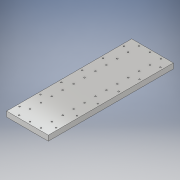
# Autodesk Inventor part: AlTop
Saved by Autodesk Inventor 2019.4 (Build 234330000, 330)
## iProperties
Created: 2020-04-27
Part Number: AlTop
Material: Generic
Document SubType Name: Modeling
Designer: Ed
Density: 1 g/cm^3
Appearance: Default
Author: Ed
Autodesk Inventor part; units mm, degrees
ref_plane "YZ Plane" through (0, 0, 0) normal (1, 0, 0) x (0, 1, 0)
ref_plane "XZ Plane" through (0, 0, 0) normal (0, 1, 0) x (-1, 0, 0)
ref_plane "XY Plane" through (0, 0, 0) normal (0, 0, 1) x (1, 0, 0)
sketch "Sketch1" plane through (0, 0, 0) normal (0, 1, 0) x (-1, 0, 0)
  arc A0 (49.1631, 298.6655) -> (49.149, 298.45) centre (50.8, 298.45) ccw
  arc A1 (49.149, 298.45) -> (52.3947, 298.0227) centre (50.8, 298.45) ccw
  arc A2 (52.3947, 298.0227) -> (52.451, 298.45) centre (50.8, 298.45) ccw
  arc A3 (52.451, 298.45) -> (49.2053, 298.8773) centre (50.8, 298.45) ccw
  arc A4 (49.2053, 298.8773) -> (49.1631, 298.6655) centre (50.8, 298.45) ccw
  arc A5 (22.7572, 297.5315) -> (22.9626, 297.2813) centre (24.13, 298.4487) ccw
  arc A6 (22.9626, 297.2813) -> (25.781, 298.4487) centre (24.13, 298.4487) ccw
  arc A7 (25.781, 298.4487) -> (22.5353, 298.876) centre (24.13, 298.4487) ccw
  arc A8 (22.5353, 298.876) -> (22.479, 298.4487) centre (24.13, 298.4487) ccw
  arc A9 (22.479, 298.4487) -> (22.7572, 297.5315) centre (24.13, 298.4487) ccw
  arc A10 (7.7798, 278.5745) -> (8.001, 279.4) centre (6.35, 279.4) ccw
  arc A11 (8.001, 279.4) -> (7.5174, 280.5674) centre (6.35, 279.4) ccw
  arc A12 (7.5174, 280.5674) -> (6.35, 281.051) centre (6.35, 279.4) ccw
  arc A13 (6.35, 281.051) -> (5.1826, 280.5674) centre (6.35, 279.4) ccw
  arc A14 (5.1826, 280.5674) -> (4.699, 279.4) centre (6.35, 279.4) ccw
  arc A15 (4.699, 279.4) -> (7.7798, 278.5745) centre (6.35, 279.4) ccw
  arc A16 (23.8079, 270.275) -> (24.13, 270.2433) centre (24.13, 271.8943) ccw
  arc A17 (24.13, 270.2433) -> (25.781, 271.8943) centre (24.13, 271.8943) ccw
  arc A18 (25.781, 271.8943) -> (23.3045, 273.3241) centre (24.13, 271.8943) ccw
  arc A19 (23.3045, 273.3241) -> (22.7002, 272.7198) centre (24.13, 271.8943) ccw
  arc A20 (22.7002, 272.7198) -> (22.479, 271.8943) centre (24.13, 271.8943) ccw
  arc A21 (22.479, 271.8943) -> (23.8079, 270.275) centre (24.13, 271.8943) ccw
  arc A22 (22.7002, 244.5144) -> (25.781, 245.3399) centre (24.13, 245.3399) ccw
  arc A23 (25.781, 245.3399) -> (24.4521, 246.9591) centre (24.13, 245.3399) ccw
  arc A24 (24.4521, 246.9591) -> (23.7027, 246.9346) centre (24.13, 245.3399) ccw
  arc A25 (23.7027, 246.9346) -> (22.479, 245.3399) centre (24.13, 245.3399) ccw
  arc A26 (22.479, 245.3399) -> (22.7002, 244.5144) centre (24.13, 245.3399) ccw
  arc A27 (7.7798, 227.7745) -> (8.001, 228.6) centre (6.35, 228.6) ccw
  arc A28 (8.001, 228.6) -> (7.5174, 229.7674) centre (6.35, 228.6) ccw
  arc A29 (7.5174, 229.7674) -> (6.35, 230.251) centre (6.35, 228.6) ccw
  arc A30 (6.35, 230.251) -> (4.699, 228.6) centre (6.35, 228.6) ccw
  arc A31 (4.699, 228.6) -> (7.7798, 227.7745) centre (6.35, 228.6) ccw
  arc A32 (23.7027, 217.1907) -> (25.781, 218.7854) centre (24.13, 218.7854) ccw
  arc A33 (25.781, 218.7854) -> (23.7027, 220.3802) centre (24.13, 218.7854) ccw
  arc A34 (23.7027, 220.3802) -> (22.8202, 219.7905) centre (24.13, 218.7854) ccw
  arc A35 (22.8202, 219.7905) -> (22.479, 218.7854) centre (24.13, 218.7854) ccw
  arc A36 (22.479, 218.7854) -> (23.7027, 217.1907) centre (24.13, 218.7854) ccw
  arc A37 (22.7002, 191.4055) -> (25.781, 192.231) centre (24.13, 192.231) ccw
  arc A38 (25.781, 192.231) -> (24.4521, 193.8503) centre (24.13, 192.231) ccw
  arc A39 (24.4521, 193.8503) -> (23.7027, 193.8258) centre (24.13, 192.231) ccw
  arc A40 (23.7027, 193.8258) -> (22.479, 192.231) centre (24.13, 192.231) ccw
  arc A41 (22.479, 192.231) -> (22.7002, 191.4055) centre (24.13, 192.231) ccw
  arc A42 (7.5174, 176.6326) -> (8.001, 177.8) centre (6.35, 177.8) ccw
  arc A43 (8.001, 177.8) -> (7.7228, 178.7172) centre (6.35, 177.8) ccw
  arc A44 (7.7228, 178.7172) -> (6.35, 179.451) centre (6.35, 177.8) ccw
  arc A45 (6.35, 179.451) -> (4.699, 177.8) centre (6.35, 177.8) ccw
  arc A46 (4.699, 177.8) -> (7.5174, 176.6326) centre (6.35, 177.8) ccw
  arc A47 (23.7027, 164.0818) -> (25.781, 165.6766) centre (24.13, 165.6766) ccw
  arc A48 (25.781, 165.6766) -> (24.13, 167.3276) centre (24.13, 165.6766) ccw
  arc A49 (24.13, 167.3276) -> (22.9626, 166.844) centre (24.13, 165.6766) ccw
  arc A50 (22.9626, 166.844) -> (22.479, 165.6766) centre (24.13, 165.6766) ccw
  arc A51 (22.479, 165.6766) -> (23.7027, 164.0818) centre (24.13, 165.6766) ccw
  arc A52 (22.7002, 138.2966) -> (25.781, 139.1221) centre (24.13, 139.1221) ccw
  arc A53 (25.781, 139.1221) -> (24.4521, 140.7414) centre (24.13, 139.1221) ccw
  arc A54 (24.4521, 140.7414) -> (24.3723, 140.7553) centre (24.13, 139.1221) ccw
  arc A55 (24.3723, 140.7553) -> (24.13, 140.7731) centre (24.13, 139.1221) ccw
  arc A56 (24.13, 140.7731) -> (22.479, 139.1221) centre (24.13, 139.1221) ccw
  arc A57 (22.479, 139.1221) -> (22.7002, 138.2966) centre (24.13, 139.1221) ccw
  arc A58 (7.5174, 125.8326) -> (8.001, 127) centre (6.35, 127) ccw
  arc A59 (8.001, 127) -> (7.7228, 127.9172) centre (6.35, 127) ccw
  arc A60 (7.7228, 127.9172) -> (6.35, 128.651) centre (6.35, 127) ccw
  arc A61 (6.35, 128.651) -> (4.699, 127) centre (6.35, 127) ccw
  arc A62 (4.699, 127) -> (7.5174, 125.8326) centre (6.35, 127) ccw
  arc A63 (23.7027, 110.973) -> (25.781, 112.5677) centre (24.13, 112.5677) ccw
  arc A64 (25.781, 112.5677) -> (24.13, 114.2187) centre (24.13, 112.5677) ccw
  arc A65 (24.13, 114.2187) -> (22.9626, 113.7352) centre (24.13, 112.5677) ccw
  arc A66 (22.9626, 113.7352) -> (22.479, 112.5677) centre (24.13, 112.5677) ccw
  arc A67 (22.479, 112.5677) -> (23.7027, 110.973) centre (24.13, 112.5677) ccw
  arc A68 (22.5353, 85.586) -> (25.781, 86.0133) centre (24.13, 86.0133) ccw
  arc A69 (25.781, 86.0133) -> (24.4521, 87.6326) centre (24.13, 86.0133) ccw
  arc A70 (24.4521, 87.6326) -> (24.3723, 87.6464) centre (24.13, 86.0133) ccw
  arc A71 (24.3723, 87.6464) -> (24.13, 87.6643) centre (24.13, 86.0133) ccw
  arc A72 (24.13, 87.6643) -> (22.479, 86.0133) centre (24.13, 86.0133) ccw
  arc A73 (22.479, 86.0133) -> (22.5353, 85.586) centre (24.13, 86.0133) ccw
  arc A74 (7.5174, 75.0326) -> (8.001, 76.2) centre (6.35, 76.2) ccw
  arc A75 (8.001, 76.2) -> (7.8753, 76.8318) centre (6.35, 76.2) ccw
  arc A76 (7.8753, 76.8318) -> (6.35, 77.851) centre (6.35, 76.2) ccw
  arc A77 (6.35, 77.851) -> (4.699, 76.2) centre (6.35, 76.2) ccw
  arc A78 (4.699, 76.2) -> (7.5174, 75.0326) centre (6.35, 76.2) ccw
  arc A79 (23.7027, 57.8641) -> (25.781, 59.4589) centre (24.13, 59.4589) ccw
  arc A80 (25.781, 59.4589) -> (24.13, 61.1099) centre (24.13, 59.4589) ccw
  arc A81 (24.13, 61.1099) -> (23.2128, 60.8316) centre (24.13, 59.4589) ccw
  arc A82 (23.2128, 60.8316) -> (22.479, 59.4589) centre (24.13, 59.4589) ccw
  arc A83 (22.479, 59.4589) -> (23.7027, 57.8641) centre (24.13, 59.4589) ccw
  arc A84 (22.5353, 32.4771) -> (25.781, 32.9044) centre (24.13, 32.9044) ccw
  arc A85 (25.781, 32.9044) -> (24.4521, 34.5237) centre (24.13, 32.9044) ccw
  arc A86 (24.4521, 34.5237) -> (24.3723, 34.5376) centre (24.13, 32.9044) ccw
  arc A87 (24.3723, 34.5376) -> (24.13, 34.5554) centre (24.13, 32.9044) ccw
  arc A88 (24.13, 34.5554) -> (22.479, 32.9044) centre (24.13, 32.9044) ccw
  arc A89 (22.479, 32.9044) -> (22.5353, 32.4771) centre (24.13, 32.9044) ccw
  arc A90 (7.1755, 23.9702) -> (8.001, 25.4) centre (6.35, 25.4) ccw
  arc A91 (8.001, 25.4) -> (7.9299, 25.8793) centre (6.35, 25.4) ccw
  arc A92 (7.9299, 25.8793) -> (7.8753, 26.0318) centre (6.35, 25.4) ccw
  arc A93 (7.8753, 26.0318) -> (6.35, 27.051) centre (6.35, 25.4) ccw
  arc A94 (6.35, 27.051) -> (4.699, 25.4) centre (6.35, 25.4) ccw
  arc A95 (4.699, 25.4) -> (7.1755, 23.9702) centre (6.35, 25.4) ccw
  arc A96 (25.7247, 5.9227) -> (25.781, 6.35) centre (24.13, 6.35) ccw
  arc A97 (25.781, 6.35) -> (24.13, 8.001) centre (24.13, 6.35) ccw
  arc A98 (24.13, 8.001) -> (23.2128, 7.7228) centre (24.13, 6.35) ccw
  arc A99 (23.2128, 7.7228) -> (22.479, 6.35) centre (24.13, 6.35) ccw
  arc A100 (22.479, 6.35) -> (25.7247, 5.9227) centre (24.13, 6.35) ccw
  arc A101 (52.4369, 6.1345) -> (52.451, 6.35) centre (50.8, 6.35) ccw
  arc A102 (52.451, 6.35) -> (50.3727, 7.9447) centre (50.8, 6.35) ccw
  arc A103 (50.3727, 7.9447) -> (49.149, 6.35) centre (50.8, 6.35) ccw
  arc A104 (49.149, 6.35) -> (52.3947, 5.9227) centre (50.8, 6.35) ccw
  arc A105 (52.3947, 5.9227) -> (52.4369, 6.1345) centre (50.8, 6.35) ccw
  arc A106 (78.7462, 7.3974) -> (77.0427, 7.9447) centre (77.47, 6.35) ccw
  arc A107 (77.0427, 7.9447) -> (75.819, 6.35) centre (77.47, 6.35) ccw
  arc A108 (75.819, 6.35) -> (79.121, 6.35) centre (77.47, 6.35) ccw
  arc A109 (79.121, 6.35) -> (78.7462, 7.3974) centre (77.47, 6.35) ccw
  arc A110 (93.8624, 26.2947) -> (93.6866, 25.9307) centre (95.25, 25.4) ccw
  arc A111 (93.6866, 25.9307) -> (93.599, 25.4) centre (95.25, 25.4) ccw
  arc A112 (93.599, 25.4) -> (94.0826, 24.2326) centre (95.25, 25.4) ccw
  arc A113 (94.0826, 24.2326) -> (96.901, 25.4) centre (95.25, 25.4) ccw
  arc A114 (96.901, 25.4) -> (94.8227, 26.9947) centre (95.25, 25.4) ccw
  arc A115 (94.8227, 26.9947) -> (93.8624, 26.2947) centre (95.25, 25.4) ccw
  arc A116 (77.7921, 34.5237) -> (77.0427, 34.4992) centre (77.47, 32.9044) ccw
  arc A117 (77.0427, 34.4992) -> (75.819, 32.9044) centre (77.47, 32.9044) ccw
  arc A118 (75.819, 32.9044) -> (78.8998, 32.0789) centre (77.47, 32.9044) ccw
  arc A119 (78.8998, 32.0789) -> (79.121, 32.9044) centre (77.47, 32.9044) ccw
  arc A120 (79.121, 32.9044) -> (77.7921, 34.5237) centre (77.47, 32.9044) ccw
  arc A121 (78.7462, 60.5062) -> (77.0427, 61.0536) centre (77.47, 59.4589) ccw
  arc A122 (77.0427, 61.0536) -> (75.819, 59.4589) centre (77.47, 59.4589) ccw
  arc A123 (75.819, 59.4589) -> (77.0427, 57.8641) centre (77.47, 59.4589) ccw
  arc A124 (77.0427, 57.8641) -> (79.121, 59.4589) centre (77.47, 59.4589) ccw
  arc A125 (79.121, 59.4589) -> (78.7462, 60.5062) centre (77.47, 59.4589) ccw
  arc A126 (93.9402, 77.2051) -> (93.599, 76.2) centre (95.25, 76.2) ccw
  arc A127 (93.599, 76.2) -> (94.0826, 75.0326) centre (95.25, 76.2) ccw
  arc A128 (94.0826, 75.0326) -> (96.901, 76.2) centre (95.25, 76.2) ccw
  arc A129 (96.901, 76.2) -> (94.8227, 77.7947) centre (95.25, 76.2) ccw
  arc A130 (94.8227, 77.7947) -> (93.9402, 77.2051) centre (95.25, 76.2) ccw
  arc A131 (77.7921, 87.6326) -> (77.0427, 87.608) centre (77.47, 86.0133) ccw
  arc A132 (77.0427, 87.608) -> (75.819, 86.0133) centre (77.47, 86.0133) ccw
  arc A133 (75.819, 86.0133) -> (78.8998, 85.1878) centre (77.47, 86.0133) ccw
  arc A134 (78.8998, 85.1878) -> (79.121, 86.0133) centre (77.47, 86.0133) ccw
  arc A135 (79.121, 86.0133) -> (77.7921, 87.6326) centre (77.47, 86.0133) ccw
  arc A136 (78.9507, 113.2979) -> (77.0427, 114.1625) centre (77.47, 112.5677) ccw
  arc A137 (77.0427, 114.1625) -> (75.819, 112.5677) centre (77.47, 112.5677) ccw
  arc A138 (75.819, 112.5677) -> (77.0427, 110.973) centre (77.47, 112.5677) ccw
  arc A139 (77.0427, 110.973) -> (79.121, 112.5677) centre (77.47, 112.5677) ccw
  arc A140 (79.121, 112.5677) -> (78.9507, 113.2979) centre (77.47, 112.5677) ccw
  arc A141 (94.0826, 128.1674) -> (93.599, 127) centre (95.25, 127) ccw
  arc A142 (93.599, 127) -> (93.8202, 126.1745) centre (95.25, 127) ccw
  arc A143 (93.8202, 126.1745) -> (96.901, 127) centre (95.25, 127) ccw
  arc A144 (96.901, 127) -> (94.4245, 128.4298) centre (95.25, 127) ccw
  arc A145 (94.4245, 128.4298) -> (94.0826, 128.1674) centre (95.25, 127) ccw
  arc A146 (77.578, 140.7696) -> (76.6445, 140.552) centre (77.47, 139.1222) ccw
  arc A147 (76.6445, 140.552) -> (75.819, 139.1221) centre (77.47, 139.1222) ccw
  arc A148 (75.819, 139.1221) -> (78.6374, 137.9547) centre (77.47, 139.1222) ccw
  arc A149 (78.6374, 137.9547) -> (79.121, 139.1221) centre (77.47, 139.1222) ccw
  arc A150 (79.121, 139.1221) -> (77.8973, 140.7169) centre (77.47, 139.1222) ccw
  arc A151 (77.8973, 140.7169) -> (77.578, 140.7696) centre (77.47, 139.1222) ccw
  arc A152 (78.9953, 166.3084) -> (78.8998, 166.5021) centre (77.47, 165.6766) ccw
  arc A153 (78.8998, 166.5021) -> (76.6445, 167.1064) centre (77.47, 165.6766) ccw
  arc A154 (76.6445, 167.1064) -> (75.819, 165.6766) centre (77.47, 165.6766) ccw
  arc A155 (75.819, 165.6766) -> (77.0427, 164.0818) centre (77.47, 165.6766) ccw
  arc A156 (77.0427, 164.0818) -> (79.121, 165.6766) centre (77.47, 165.6766) ccw
  arc A157 (79.121, 165.6766) -> (78.9953, 166.3084) centre (77.47, 165.6766) ccw
  arc A158 (94.1614, 179.0413) -> (94.0826, 178.9674) centre (95.25, 177.8) ccw
  arc A159 (94.0826, 178.9674) -> (93.599, 177.8) centre (95.25, 177.8) ccw
  arc A160 (93.599, 177.8) -> (93.8202, 176.9745) centre (95.25, 177.8) ccw
  arc A161 (93.8202, 176.9745) -> (96.901, 177.8) centre (95.25, 177.8) ccw
  arc A162 (96.901, 177.8) -> (94.4245, 179.2298) centre (95.25, 177.8) ccw
  arc A163 (94.4245, 179.2298) -> (94.1614, 179.0413) centre (95.25, 177.8) ccw
  arc A164 (77.578, 193.8785) -> (76.6445, 193.6608) centre (77.47, 192.231) ccw
  arc A165 (76.6445, 193.6608) -> (75.819, 192.231) centre (77.47, 192.231) ccw
  arc A166 (75.819, 192.231) -> (78.6374, 191.0636) centre (77.47, 192.231) ccw
  arc A167 (78.6374, 191.0636) -> (79.121, 192.231) centre (77.47, 192.231) ccw
  arc A168 (79.121, 192.231) -> (77.8973, 193.8258) centre (77.47, 192.231) ccw
  arc A169 (77.8973, 193.8258) -> (77.578, 193.8785) centre (77.47, 192.231) ccw
  arc A170 (79.0499, 219.2647) -> (76.3026, 219.9529) centre (77.47, 218.7854) ccw
  arc A171 (76.3026, 219.9529) -> (75.819, 218.7854) centre (77.47, 218.7854) ccw
  arc A172 (75.819, 218.7854) -> (77.0427, 217.1907) centre (77.47, 218.7854) ccw
  arc A173 (77.0427, 217.1907) -> (79.121, 218.7854) centre (77.47, 218.7854) ccw
  arc A174 (79.121, 218.7854) -> (79.0499, 219.2647) centre (77.47, 218.7854) ccw
  arc A175 (94.0826, 229.7674) -> (93.599, 228.6) centre (95.25, 228.6) ccw
  arc A176 (93.599, 228.6) -> (93.8202, 227.7745) centre (95.25, 228.6) ccw
  arc A177 (93.8202, 227.7745) -> (96.901, 228.6) centre (95.25, 228.6) ccw
  arc A178 (96.901, 228.6) -> (94.0826, 229.7674) centre (95.25, 228.6) ccw
  arc A179 (77.6318, 246.9829) -> (76.3026, 246.5073) centre (77.47, 245.3399) ccw
  arc A180 (76.3026, 246.5073) -> (75.819, 245.3399) centre (77.47, 245.3399) ccw
  arc A181 (75.819, 245.3399) -> (78.6374, 244.1724) centre (77.47, 245.3399) ccw
  arc A182 (78.6374, 244.1724) -> (79.121, 245.3399) centre (77.47, 245.3399) ccw
  arc A183 (79.121, 245.3399) -> (77.6318, 246.9829) centre (77.47, 245.3399) ccw
  arc A184 (79.0612, 272.3346) -> (79.0152, 272.4759) centre (77.47, 271.8943) ccw
  arc A185 (79.0152, 272.4759) -> (75.8753, 272.3216) centre (77.47, 271.8943) ccw
  arc A186 (75.8753, 272.3216) -> (75.819, 271.8943) centre (77.47, 271.8943) ccw
  arc A187 (75.819, 271.8943) -> (77.0427, 270.2996) centre (77.47, 271.8943) ccw
  arc A188 (77.0427, 270.2996) -> (79.121, 271.8943) centre (77.47, 271.8943) ccw
  arc A189 (79.121, 271.8943) -> (79.0612, 272.3346) centre (77.47, 271.8943) ccw
  arc A190 (94.3328, 280.7728) -> (93.6553, 279.8273) centre (95.25, 279.4) ccw
  arc A191 (93.6553, 279.8273) -> (93.599, 279.4) centre (95.25, 279.4) ccw
  arc A192 (93.599, 279.4) -> (93.6553, 278.9727) centre (95.25, 279.4) ccw
  arc A193 (93.6553, 278.9727) -> (96.901, 279.4) centre (95.25, 279.4) ccw
  arc A194 (96.901, 279.4) -> (94.3328, 280.7728) centre (95.25, 279.4) ccw
  arc A195 (79.0152, 299.0303) -> (75.8753, 298.876) centre (77.47, 298.4487) ccw
  arc A196 (75.8753, 298.876) -> (75.819, 298.4487) centre (77.47, 298.4487) ccw
  arc A197 (75.819, 298.4487) -> (78.2955, 297.0189) centre (77.47, 298.4487) ccw
  arc A198 (78.2955, 297.0189) -> (79.121, 298.4487) centre (77.47, 298.4487) ccw
  arc A199 (79.121, 298.4487) -> (79.0152, 299.0303) centre (77.47, 298.4487) ccw
  line L0 (101.6, 0) -> (101.6, 304.8)
  line L1 (0, 0) -> (101.6, 0)
  line L2 (0, 304.8) -> (0, 0)
  line L3 (101.6, 304.8) -> (0, 304.8)
  constraints: 400 point on circle, 200 centre point, 37 equal radius, 8 end point, 2 perpendicular, 1 parallel
extrude "Extrusion1" add sketch "Sketch1" along normal blind 12.7
body "Solid1"
